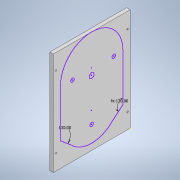
# Autodesk Inventor part: front plate
Saved by Autodesk Inventor 2020.3 (Build 243373000, 373)
## iProperties
Created: 2020-08-09
Part Number: front plate
Material: Generic
Document SubType Name: Modeling
Designer: joesp
Density: 1 g/cm^3
Appearance: Default
Author: joesp
Autodesk Inventor part; units mm, degrees
ref_plane "YZ Plane" through (0, 0, 0) normal (1, 0, 0) x (0, 1, 0)
ref_plane "XZ Plane" through (0, 0, 0) normal (0, 1, 0) x (-1, 0, 0)
ref_plane "XY Plane" through (0, 0, 0) normal (0, 0, 1) x (1, 0, 0)
sketch "Sketch1" plane through (0, 0, 0) normal (1, 0, 0) x (0, 1, 0)
  line L0 (0, 0) -> (147, 0)
  line L1 (147, 0) -> (147, 110)
  line L2 (147, 110) -> (0, 110)
  line L3 (0, 110) -> (0, 0)
  circle A0 centre (124.75, 106.25) radius 1
  circle A1 centre (124.75, 3.75) radius 1
  circle A2 centre (22.25, 3.75) radius 1
  circle A3 centre (22.25, 106.25) radius 1
  dimension "d0" = 102.5
  dimension "d1" = 102.5
  dimension "d2" = 2
  dimension "d3" = 110
  dimension "d4" = 147
  dimension "d5" = 22.25
  dimension "d6" = 22.25
  dimension "d7" = 3.75
  dimension "d8" = 3.75
  constraints: 8 end point, 4 centre point, 3 equal radius, 2 horizontal alignment, 2 parallel, 2 vertical alignment, 1 horizontal, 1 perpendicular
  measures "d0" distance of A1.centre A0.centre
  measures "d1" distance of A3.centre A0.centre
  measures "d2" diameter of A0
  measures "d3" distance of L0.end L1.end
  measures "d4" distance of L1.end L2.end
  measures "d5" distance from line of L1 A0.centre
  measures "d6" distance from line of L3 A3.centre
  measures "d7" distance from line of L2 A0.centre
  measures "d8" distance from line of L0 A1.centre
extrude "Extrusion1" add sketch "Sketch1" along normal blind 5
sketch "Sketch4" plane through (5, 0, 0) normal (1, 0, 0) x (0, 0, -1)
  circle A0 centre (-23.7023, 101.2875) radius 2.5388
  circle A1 centre (-82.8153, 101.2875) radius 2.5388
  circle A2 centre (-55.3839, 32.6302) radius 2.5388
  circle A3 centre (-55.3839, 93.3622) radius 3.4833
  line L0 (-100.0987, 102.591) -> (-100.0987, 34.6668)
  line L1 (-100.0987, 34.6668) -> (-84.8032, 21.8323)
  arc A4 (-84.8032, 21.8323) -> (-25.9646, 21.8323) centre (-55.3839, 50.0088) ccw
  line L2 (-25.9646, 21.8323) -> (-10.6691, 34.6668)
  line L3 (-10.6691, 34.6668) -> (-10.6691, 102.591)
  arc A5 (-10.6691, 102.591) -> (-100.0987, 102.591) centre (-55.3839, 102.591) ccw
  point P0 (0, 0)
  dimension "d36" = 130
  dimension "d37" = 130
  constraints: 8 end point, 6 centre point, 4 point on circle, 3 vertical alignment, 2 equal length, 2 equal radius, 2 horizontal alignment, 2 vertical
  measures "d36" angle of L0 L1
  measures "d37" angle of L3 L2
equation "\"d1\" = d0"
equation "\"d5\" = d6"
equation "\"d7\" = d8"
equation "\"d37\" = d36"
body "Solid1"
